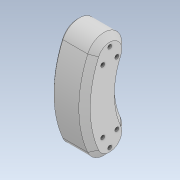
# Autodesk Inventor part: thigh_link
Saved by Autodesk Inventor 2020 (Build 240168000, 168)
## iProperties
Created: 2020-12-22
Part Number: thigh_link
Material: Generic
Document SubType Name: Modeling
Designer: DELL
Density: 1 g/cm^3
Appearance: Default
Author: DELL
Autodesk Inventor part; units mm, degrees
ref_plane "YZ Plane" through (0, 0, 0) normal (1, 0, 0) x (0, 1, 0)
ref_plane "XZ Plane" through (0, 0, 0) normal (0, 1, 0) x (-1, 0, 0)
ref_plane "XY Plane" through (0, 0, 0) normal (0, 0, 1) x (1, 0, 0)
sketch "Sketch1" plane through (0, 0, 0) normal (1, 0, 0) x (0, 1, 0)
  circle A0 centre (0, 0) radius 11.5 construction
  circle A1 centre (-100, 0) radius 11.5 construction
  line L0 (0, 0) -> (-100, 0) construction
  circle A2 centre (11.5, 0) radius 1.65
  circle A3 centre (-5.75, 9.9593) radius 1.65
  circle A4 centre (-5.75, -9.9593) radius 1.65
  line L1 (0, 0) -> (-5.75, 9.9593) construction
  line L2 (0, 0) -> (-5.75, -9.9593) construction
  line L3 (0, 11.5) -> (0, -11.5) construction
  circle A5 centre (0, 0) radius 9.715 construction
  circle A6 centre (-9.715, 0) radius 2
  circle A7 centre (4.8575, 8.4134) radius 2
  circle A8 centre (4.8575, -8.4134) radius 2
  line L4 (0, 0) -> (5.75, 9.9593) construction
  line L5 (0, 0) -> (5.75, -9.9593) construction
  circle A9 centre (0, 0) radius 25
  line L6 (-50, 45.5759) -> (-50, -45.5759) construction
  circle A10 centre (-111.5, 0) radius 1.65
  circle A11 centre (-94.25, 9.9593) radius 1.65
  circle A12 centre (-94.25, -9.9593) radius 1.65
  circle A13 centre (-90.285, 0) radius 2
  circle A14 centre (-104.8575, 8.4134) radius 2
  circle A15 centre (-104.8575, -8.4134) radius 2
  circle A16 centre (-100, 0) radius 25
  arc A17 (10, 22.9129) -> (-110, 22.9129) centre (-50, -114.5644) ccw
  arc A18 (-10, -22.9129) -> (-90, -22.9129) centre (-50, -114.5644) ccw
  circle A19 centre (11.5, 0) radius 2.75
  circle A20 centre (-5.75, 9.9593) radius 2.75
  circle A21 centre (-5.75, -9.9593) radius 2.75
  circle A22 centre (-111.5, 0) radius 2.75
  circle A23 centre (-94.25, 9.9593) radius 2.75
  circle A24 centre (-94.25, -9.9593) radius 2.75
  point P0 (-50, 0)
  dimension "d0" = 23
  dimension "d1" = 100
  dimension "d2" = 3.3
  dimension "d3" = 30
  dimension "d4" = 30
  dimension "d5" = 19.43
  dimension "d6" = 4
  dimension "d7" = 30
  dimension "d8" = 50
  dimension "d9" = 200
  dimension "d12" = 5.5
  dimension "d23" = 150
  constraints: 24 centre point, 14 end point, 11 point on circle, 10 symmetric about line, 6 coincident, 6 equal radius, 4 midpoint, 4 point on line, 2 tangent, 2 vertical, 1 horizontal, 1 horizontal alignment, 21 other
  measures "d1" distance of L0.end point (0, 0)
  measures "d2" diameter of A2
  measures "d3" angle of L3 L1
  measures "d4" angle of L3 L2
  measures "d5" diameter of A5
  measures "d6" diameter of A7
  measures "d7" angle of L3 L4
  measures "d8" diameter of A9
  measures "d9" diameter of A18
  measures "d12" diameter of A19
  measures "d23" radius of A17
extrude "Extrusion1" add sketch "Sketch1" against normal blind 45 contours A6 | A7 | A8 | A9 | A9 A18 A16 A17 | A16 | A13 | A14 | A15 | A19 | A20 | A21 | A22 | A23 | A24
extrude "Extrusion2" cut sketch "Sketch1" against normal blind 35 contours A19 | A20 | A21 | A22 | A23 | A24
extrude "Extrusion3" cut sketch "Sketch1" along normal blind 5 from surface at -45 contours A6 | A7 | A8 | A13 | A14 | A15
chamfer "Chamfer1" distance 8 angle 45 4 edges at (0, 22.9129, -10) (0, -50, 35.4356) (0, -122.9129, -10) (0, -50, -14.5644)
chamfer "Chamfer2" distance 2 angle 45 4 edges at (-45, 22.9129, -10) (-45, -50, -14.5644) (-45, -122.9129, -10) (-45, -50, 35.4356)
equation "\"d1\" = thigh_length"
equation "\"thigh_length\" = 100"
body "Solid1"
